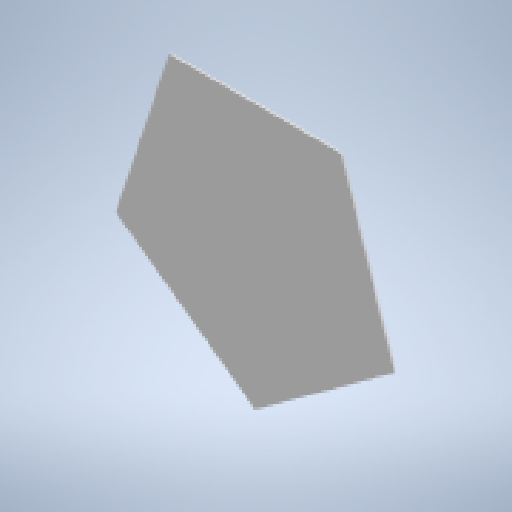
# Autodesk Inventor part: Pentagono
Saved by Autodesk Inventor 2024.2 (Build 282272000, 272)
## iProperties
Created: 2024-04-24
Part Number: Pentagono
Material: Genérico
Document SubType Name: Modeling
Designer: sergi
Density: 1 g/cm^3
Appearance: Valor por defecto
Author: sergi
Autodesk Inventor part; units mm, degrees
ref_plane "YZ Plane" through (0, 0, 0) normal (1, 0, 0) x (0, 1, 0)
ref_plane "XZ Plane" through (0, 0, 0) normal (0, 1, 0) x (-1, 0, 0)
ref_plane "XY Plane" through (0, 0, 0) normal (0, 0, 1) x (1, 0, 0)
sketch "Boceto1" plane through (0, 0, 0) normal (0, 0, 1) x (1, 0, 0)
  line L0 (78.56, -21.6086) -> (46.5862, 76.7964) projected
  line L1 (82.0867, -22.7545) -> (78.56, -21.6086) projected
  line L2 (82.0867, -22.7545) -> (48.7659, 79.7964) projected
  line L3 (46.5862, 76.7964) -> (48.7659, 79.7964) projected
  line L4 (-5.1483, -82.4262) -> (78.56, -21.6086) projected
  line L5 (-5.1483, -86.1344) -> (-5.1483, -82.4262) projected
  line L6 (-5.1483, -86.1344) -> (82.0867, -22.7545) projected
  line L7 (78.56, -21.6086) -> (82.0867, -22.7545) projected
  line L8 (-88.8566, -21.6086) -> (-5.1483, -82.4262) projected
  line L9 (-88.8566, -21.6086) -> (-92.3834, -22.7545) projected
  line L10 (-5.1483, -86.1344) -> (-92.3834, -22.7545) projected
  line L11 (-5.1483, -86.1344) -> (-5.1483, -82.4262) projected
  line L12 (-56.8829, 76.7964) -> (-88.8566, -21.6086) projected
  line L13 (-59.0626, 79.7964) -> (-56.8829, 76.7964) projected
  line L14 (-59.0626, 79.7964) -> (-92.3834, -22.7545) projected
  line L15 (-88.8566, -21.6086) -> (-92.3834, -22.7545) projected
  line L16 (46.5862, 76.7964) -> (-56.8829, 76.7964) projected
  line L17 (48.7659, 79.7964) -> (46.5862, 76.7964) projected
  line L18 (48.7659, 79.7964) -> (-59.0626, 79.7964) projected
  line L19 (-56.8829, 76.7964) -> (-59.0626, 79.7964) projected
  circle A0 centre (-5.1483, 5.5899) radius 71.2065
  line L20 (-92.3834, -22.7545) -> (-59.0626, 79.7964)
  line L21 (-59.0626, 79.7964) -> (48.7659, 79.7964)
  line L22 (48.7659, 79.7964) -> (82.0867, -22.7545)
  line L23 (82.0867, -22.7545) -> (-5.1483, -86.1344)
  line L24 (-5.1483, -86.1344) -> (-92.3834, -22.7545)
  line L25 (-5.1483, -85.5164) -> (81.4989, -22.5635)
  line L26 (81.4989, -22.5635) -> (48.4026, 79.2964)
  line L27 (48.4026, 79.2964) -> (-58.6993, 79.2964)
  line L28 (-58.6993, 79.2964) -> (-91.7956, -22.5635)
  line L29 (-91.7956, -22.5635) -> (-5.1483, -85.5164)
  point P0 (0, 0)
  point P1 (-5.1483, 5.5899)
  dimension "d0" = 0.5
  constraints: 20 end point, 3 tangent, 1 centre point, 15 other
  measures "d0" distance between parallel lines of L23 L25
extrude "Extrusión1" add sketch "Boceto1" along normal blind 1.2
